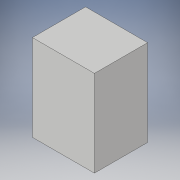
# Autodesk Inventor part: SouthWestWallBlock
Saved by Autodesk Inventor 2018 (Build 220112000, 112)
## iProperties
Created: 2019-04-28
Part Number: SouthWestWallBlock
Material: Generic
Document SubType Name: Modeling
Designer: snipe
Density: 1 g/cm^3
Appearance: Default
Author: snipe
Autodesk Inventor part; units mm, degrees
ref_plane "YZ Plane" through (0, 0, 0) normal (1, 0, 0) x (0, 1, 0)
ref_plane "XZ Plane" through (0, 0, 0) normal (0, 1, 0) x (-1, 0, 0)
ref_plane "XY Plane" through (0, 0, 0) normal (0, 0, 1) x (1, 0, 0)
sketch "Sketch1" plane through (0, 0, 0) normal (0, 1, 0) x (-1, 0, 0)
  line L0 (711.2, 609.6) -> (-711.2, 609.6)
  line L1 (-711.2, 609.6) -> (-711.2, -609.6)
  line L2 (-711.2, -609.6) -> (711.2, -609.6)
  line L3 (711.2, -609.6) -> (711.2, 609.6)
  line L4 (0, -853.44) -> (0, 853.44) projected
  line L5 (-995.68, 0) -> (995.68, 0) projected
  point P0 (0, 0)
  dimension "d0" = 1422.4
  dimension "d1" = 1219.2
  constraints: 8 end point, 2 parallel, 1 horizontal, 1 perpendicular, 2 other
  measures "d0" distance of L2.end L1.end
  measures "d1" distance of L1.end L0.end
extrude "Extrusion1" add sketch "Sketch1" along normal blind 1981.2
body "Solid1"
